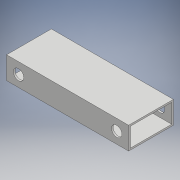
# Autodesk Inventor part: 車軸受け3
Saved by Autodesk Inventor 2018 (Build 220112000, 112)
## iProperties
Created: 2017-09-16
Part Number: 車軸受け3
Material: 一般
Document SubType Name: Modeling
Designer: mura5
Density: 1 g/cm^3
Appearance: 既定
Author: mura5
Autodesk Inventor part; units mm, degrees
ref_plane "YZ Plane" through (0, 0, 0) normal (1, 0, 0) x (0, 1, 0)
ref_plane "XZ Plane" through (0, 0, 0) normal (0, 1, 0) x (-1, 0, 0)
ref_plane "XY Plane" through (0, 0, 0) normal (0, 0, 1) x (1, 0, 0)
sketch "スケッチ1" plane through (0, 0, 0) normal (1, 0, 0) x (0, 1, 0)
  line L0 (-30, 15) -> (30, 15)
  line L1 (30, 15) -> (30, -15)
  line L2 (30, -15) -> (-30, -15)
  line L3 (-30, -15) -> (-30, 15)
  line L4 (-30, 15) -> (30, -15) construction
  line L5 (30, 15) -> (-30, -15) construction
  line L6 (27.7, 12.7) -> (-27.7, 12.7)
  line L7 (-27.7, 12.7) -> (-27.7, -12.7)
  line L8 (-27.7, -12.7) -> (27.7, -12.7)
  line L9 (27.7, -12.7) -> (27.7, 12.7)
  point P0 (0, 0)
  dimension "d0" = 60
  dimension "d1" = 30
  dimension "d2" = 2.3
  constraints: 20 end point, 4 parallel, 2 midpoint, 2 perpendicular, 1 horizontal, 3 other
  measures "d0" distance of L1.end L2.end
  measures "d1" distance of L0.end L1.end
  measures "d2" distance between parallel lines of L0 L6
extrude "押し出し1" add sketch "スケッチ1" along normal mid plane 163.5
sketch "スケッチ2" plane through (-81.75, 30, 15) normal (0, 1, 0) x (1, 0, 0)
  point P0 (81.75, 15)
  point P1 (16, 15)
  point P2 (147.5, 15)
  dimension "d5" = 65.75
  dimension "d6" = 65.75
  measures "d5" distance of point (81.75, 15) point (16, 15)
  measures "d6" distance of point (81.75, 15) point (147.5, 15)
hole "穴1" at (-65.75, 30, 0) at (65.75, 30, 0) direction (0, -1, 0) diameter 14 end through all
